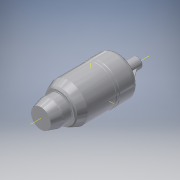
# Autodesk Inventor part: Engine
Saved by Autodesk Inventor 2019 (Build 230136000, 136)
## iProperties
Created: 2020-11-01
Part Number: Engine
Material: Generic
Document SubType Name: Modeling
Designer: rtavi
Density: 1 g/cm^3
Appearance: Smooth - White
d79: 281.000 mm
d83: 56.000 mm
d127: 4.000 mm
d128: 0.00 deg
Author: rtavi
Autodesk Inventor part; units mm, degrees
ref_plane "YZ Plane" through (0, 0, 0) normal (1, 0, 0) x (0, 1, 0)
ref_plane "XZ Plane" through (0, 0, 0) normal (0, 1, 0) x (-1, 0, 0)
ref_plane "XY Plane" through (0, 0, 0) normal (0, 0, 1) x (1, 0, 0)
sketch "Sketch3" plane through (0, 0, 0) normal (0, 1, 0) x (-1, 0, 0)
  line L0 (-148.4998, -210.0502) -> (-148.4998, 210.0502) construction
  line L1 (-148.4998, 210.0502) -> (148.4998, 210.0502) construction
  line L2 (148.4998, 210.0502) -> (148.4998, -210.0502) construction
  line L3 (148.4998, -210.0502) -> (-148.4998, -210.0502) construction
  line L4 (-278.8232, 0) -> (0, 0) construction
  line L5 (0, 0) -> (0, 323.3607) construction
  line L6 (-14.9991, -133.5139) -> (-14.9991, -118.3294)
  line L7 (-56, -69.6027) -> (-56, -30.1317)
  line L8 (-56, -30.1317) -> (-55.287, -28.2144)
  line L9 (-55.287, -28.2144) -> (-55.287, -23.6926)
  line L10 (-55.287, -23.6926) -> (-55.4718, -23.6926)
  line L11 (-55.4718, -23.6926) -> (-55.4718, -20.982)
  line L12 (-55.4718, -20.982) -> (-54.6709, -19.7868)
  line L13 (-54.6709, -19.7868) -> (-54.6709, 61.4098)
  line L14 (-54.6709, 61.4098) -> (-45.8766, 82.3346)
  line L15 (-45.8766, 82.3346) -> (-42.7179, 84.1079)
  line L16 (-42.7179, 84.1079) -> (-42.7179, 85.2162)
  line L17 (-42.7179, 85.2162) -> (-42.369, 85.2162)
  line L18 (-42.369, 85.2162) -> (-42.369, 88.0675)
  line L19 (-42.369, 88.0675) -> (-37.697, 88.0675)
  line L20 (-37.697, 88.0675) -> (-37.697, 89.6261)
  line L21 (-37.697, 89.6261) -> (-35.994, 89.6261)
  line L22 (-35.994, 89.6261) -> (-35.994, 106.9741)
  line L23 (-35.3011, 114.3761) -> (-28.055, 140.5061)
  line L24 (-28.055, 140.5061) -> (0, 140.5061)
  arc A0 (-12.1858, -137.6578) -> (-2.3721, -140.4939) centre (-0.8223, -116.7339) ccw
  arc A1 (-14.9991, -133.5139) -> (-12.1858, -137.6578) centre (-9.5817, -132.8629) ccw
  line L25 (0, -140.4939) -> (-2.3721, -140.4939)
  line L26 (0, 140.5061) -> (0, -140.4939)
  arc A2 (-35.3011, 114.3761) -> (-35.994, 106.9741) centre (-5.1555, 107.8209) ccw
  arc A3 (-56, -69.6027) -> (-40.4601, -83.9729) centre (-39.3408, -67.175) ccw
  line L27 (-40.4601, -83.9729) -> (-8.2198, -83.9729)
  line L28 (-8.2198, -83.9729) -> (-14.9991, -98.5086)
  line L29 (-14.9991, -98.5086) -> (-14.9991, -118.3294)
  dimension "d79" = 281
  dimension "d83" = 56
  constraints: 52 end point, 11 perpendicular, 8 point on circle, 4 centre point, 3 horizontal, 3 parallel, 3 vertical, 1 point on line, 1 tangent, 4 other
  measures "d79" distance of L24.end L25.start
  measures "d83" distance between parallel lines of L26 L7
revolve "Motor" add sketch "Sketch3" angle 360 about axis through (0, 0, 140.5061) along (0, 0, -1)
sketch "Sketch6" plane through (0, 0, 0) normal (0, 1, 0) x (-1, 0, 0)
  line L0 (-14.9991, -118.4458) -> (-14.9991, -98.5086)
  line L1 (-12.6573, -93.4875) -> (-23.2868, -83.9729)
  line L2 (-23.2868, -83.9729) -> (-40.5228, -83.9729)
  line L3 (-40.5228, -83.9729) -> (-14.9991, -118.4458)
  line L4 (14.9991, -98.5086) -> (-14.9991, -98.5086) projected
  line L5 (-14.9991, -98.5086) -> (-12.6573, -93.4875)
  line L6 (0, -142.1349) -> (0, 23.6892) construction
  line L7 (14.9991, -118.4458) -> (14.9991, -98.5086)
  line L8 (12.6573, -93.4875) -> (23.2868, -83.9729)
  line L9 (23.2868, -83.9729) -> (40.5228, -83.9729)
  line L10 (40.5228, -83.9729) -> (14.9991, -118.4458)
  line L11 (14.9991, -98.5086) -> (12.6573, -93.4875)
  point P0 (0, 0)
  constraints: 20 end point, 4 symmetric about line, 1 perpendicular
extrude "Motor inlet" add sketch "Sketch6" along normal mid plane 4
body "Solid1"
